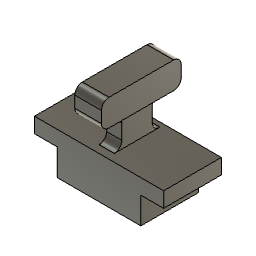
switch_emir (Autodesk Fusion 360 design; units mm, degrees)
Autodesk Fusion 360 part; units mm, degrees
sketch "Sketch1" plane through (0, 0, 0) normal (0, 1, 0) x (1, 0, 0)
  line L0 (10, -20) -> (21, -20)
  line L1 (21, -20) -> (21, -23.5)
  line L2 (21, -23.5) -> (24, -23.5)
  line L3 (24, -23.5) -> (24, -25.5)
  line L4 (24, -25.5) -> (7, -25.5)
  line L5 (7, -25.5) -> (7, -23.5)
  line L6 (7, -23.5) -> (10, -23.5)
  line L7 (10, -23.5) -> (10, -20)
  constraint horizontal L0
  constraint perpendicular L0 L1
  constraint perpendicular L1 L2
  constraint perpendicular L2 L3
  constraint perpendicular L3 L4
  constraint perpendicular L4 L5
  constraint perpendicular L5 L6
  constraint perpendicular L0 L7
extrude "Extrude1" add sketch "Sketch1" along normal blind 7.6
sketch "Sketch2" plane through (0, 0, 20) normal (0, 0, -1) x (1, 0, 0)
  line L0 (21, 0) -> (10, 0)
  line L1 (10, 0) -> (10, -7.6)
  line L2 (10, -7.6) -> (21, -7.6)
  line L3 (21, -7.6) -> (21, 0)
  line L4 (17.25, -2.05) -> (13.75, -2.05)
  line L5 (13.75, -2.05) -> (13.75, -5.55)
  line L6 (13.75, -5.55) -> (17.25, -5.55)
  line L7 (17.25, -5.55) -> (17.25, -2.05)
  line L8 (17.25, -2.05) -> (13.75, -5.55) construction
  line L9 (13.75, -2.05) -> (17.25, -5.55) construction
  point P0 (15.5, -3.8)
  dimension "d9" = 3.5
  dimension "d10" = 3.5
  constraint horizontal L4
  constraint perpendicular L4 L5
  constraint parallel L4 L6
  constraint parallel L5 L7
  constraint coincident L8 P0
  constraint coincident L9 P0
  measures "d9" distance of L5.end L6.end
  measures "d10" distance of L4.end L5.end
extrude "Extrude2" cut sketch "Sketch2" against normal blind 5 contours L4 L5 L6 L7
sketch "Sketch3" plane through (0, 0, 0) normal (0, 0, 1) x (1, 0, 0)
  line L0 (14, 0) -> (14.5, 0)
  line L1 (14.5, 0) -> (13.5, 0)
  constraint horizontal L0
  constraint parallel L0 L1
sketch "Sketch4" plane through (0, 0, 0) normal (0, -1, 0) x (1, 0, 0)
  line L0 (7, 23.5) -> (10, 23.5)
  line L1 (10, 23.5) -> (10, 20)
  line L2 (10, 20) -> (21, 20)
  line L3 (21, 20) -> (21, 23.5)
  line L4 (21, 23.5) -> (24, 23.5)
  line L5 (24, 23.5) -> (24, 25.5)
  line L6 (24, 25.5) -> (7, 25.5)
  line L7 (7, 25.5) -> (7, 23.5)
  line L8 (15.5, 25.5) -> (16.5, 25.5)
  line L9 (16.5, 25.5) -> (16.5, 29.5)
  line L10 (16.5, 29.5) -> (14.5, 29.5)
  line L11 (14.5, 29.5) -> (14.5, 25.5)
  line L12 (14.5, 25.5) -> (15.5, 25.5)
  line L13 (15.5, 29.5) -> (17.25, 29.5)
  line L14 (17.25, 29.5) -> (17.25, 33)
  line L15 (17.25, 33) -> (13.75, 33)
  line L16 (13.75, 33) -> (13.75, 29.5)
  line L17 (13.75, 29.5) -> (15.5, 29.5)
  constraint midpoint L6 L8.start
  constraint coincident L6 L8.end
  constraint perpendicular L6 L9
  constraint perpendicular L9 L10
  constraint coincident L6 L11.end
  constraint perpendicular L6 L11
  constraint midpoint L10 L13.start
  constraint parallel L10 L13
  constraint perpendicular L13 L14
  constraint perpendicular L9 L15
  constraint perpendicular L15 L16
  constraint perpendicular L16 L17
extrude "Extrude3" add sketch "Sketch4" against normal blind 4 from surface at -2 contours L6 L8 L9 L10 L11 L12 L13 L17
extrude "Extrude4" add sketch "Sketch4" against normal blind 10.5 from surface at 1.44 contours L10 L13 L14 L15 L16 L17
fillet "Fillet1" radius 1 8 edges at (15.5, -1.44, 29.5) (15.5, -1.44, 33) (15.5, 9.06, 33) (15.5, 9.06, 29.5) (15.5, 6, 29.5) (15.5, 2, 29.5) (15.5, 2, 25.5) (15.5, 6, 25.5)
